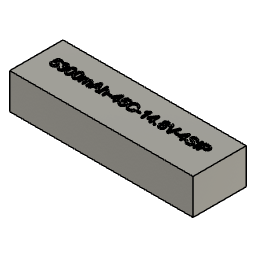
格氏电池 v2 (Autodesk Fusion 360 design; units mm, degrees)
Autodesk Fusion 360 part; units mm, degrees
sketch "草图1" plane through (0, 0, 0) normal (0, 0, 1) x (1, 0, 0)
  line L0 (0, 0) -> (155, 0)
  line L1 (155, 0) -> (155, 45)
  line L2 (155, 45) -> (0, 45)
  line L3 (0, 45) -> (0, 0)
  dimension "d1" = 155
  dimension "d2" = 45
  constraint horizontal L0
  constraint vertical L1
  constraint horizontal L2
  constraint vertical L3
  constraint coincident L0.start L3.end
  measures "d1" distance of L0.start L0.end
  measures "d2" distance of L0.start L2.end
extrude "拉伸1" add sketch "草图1" along normal blind 30 makes body 1
sketch "草图2" plane through (0, 0, 30) normal (0, 0, 1) x (-1, 0, 0)
  line L0 (0, -45) -> (0, 0)
  line L1 (0, 0) -> (-155, 0)
  line L2 (-155, 0) -> (-155, -45)
  line L3 (-155, -45) -> (0, -45)
  line L4 (-11.6459, 9.5497) -> (-154.8907, 9.5497) construction
  line L5 (-154.8907, 9.5497) -> (-154.8907, -28.8819) construction
  line L6 (-154.8907, -28.8819) -> (-11.6459, -28.8819) construction
  line L7 (-11.6459, -28.8819) -> (-11.6459, 9.5497) construction
  dimension "d5" = 8
  text T0 "5300mAh-45C-14.8V-4SIP" font "Arial" height 8 align left top in box 143.2448 x 38.4315 at (-11.6459, 9.5497) x (-1, 0) y (0, -1) spacing 1 kerned
extrude "拉伸2" add sketch "草图2" along normal blind 1 text T0 bodies 1
copy_body "实体->零部件1" bodies 1 removing the originals makes body 2 in component "Component'"
component "Component'" placed x (1, 0, 0) y (0, 1, 0) z (0, 0, 1) at (0, 0, 0)
